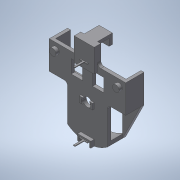
# Autodesk Inventor part: cr2032
Saved by Autodesk Inventor 2021 (Build 250183000, 183)
## iProperties
Created: 2016-08-23
Part Number: cr2032
Material: Generic
Document SubType Name: Modeling
Designer: Federico
Density: 1 g/cm^3
Appearance: Default
Author: Federico
Autodesk Inventor part; units mm, degrees
ref_plane "YZ Plane" through (0, 0, 0) normal (1, 0, 0) x (0, 1, 0)
ref_plane "XZ Plane" through (0, 0, 0) normal (0, 1, 0) x (-1, 0, 0)
ref_plane "XY Plane" through (0, 0, 0) normal (0, 0, 1) x (1, 0, 0)
sketch "Sketch1" plane through (0, 0, 0) normal (0, 1, 0) x (-1, 0, 0)
  line L0 (-2.2802, 25.7355) -> (0.7198, 25.7355)
  line L1 (0.7198, 25.7355) -> (0.7198, 20.2355)
  line L2 (0.7198, 20.2355) -> (9.2198, 20.2355)
  line L3 (9.2198, 20.2355) -> (9.2198, 11.7355)
  line L4 (9.2198, 11.7355) -> (3.7198, 11.7355)
  line L5 (3.7198, 11.7355) -> (3.7198, 0.7355)
  arc A0 (-2.2802, -1.2645) -> (3.7198, 0.7355) centre (-2.2802, 8.7355) ccw
  line L6 (-2.2802, 25.7355) -> (-2.2802, -1.2645)
  point P0 (0, 0)
  dimension "d0" = 3
  dimension "d3" = 8.5
  dimension "d4" = 5.5
  dimension "d5" = 11.5
  dimension "d6" = 6
  dimension "d9" = 27
  dimension "d10" = 11
  constraints: 14 end point, 3 parallel, 3 perpendicular, 2 point on circle, 1 centre point, 1 horizontal, 1 point on line
  measures "d0" distance of L0.start L0.end
  measures "d3" distance of L2.end L3.end
  measures "d4" distance between parallel lines of L2 L0
  measures "d5" distance from line of L3 L0.start
  measures "d6" distance from line of L6.end L5
  measures "d9" distance of L0.start L6.end
  measures "d10" distance of L4.end L5.end
extrude "base" add sketch "Sketch1" along normal blind 1
sketch "Sketch2" plane through (0, 1, 0) normal (0, 1, 0) x (1, 0, 0)
  line L0 (-0.7198, -25.7355) -> (2.2802, -25.7355) projected
  line L1 (2.2802, -25.7355) -> (2.2802, 1.2645) projected
  arc A0 (2.2802, 1.2645) -> (-3.7198, -0.7355) centre (2.2802, -8.7355) ccw projected
  line L2 (-3.7198, -0.7355) -> (-3.7198, -11.7355) projected
  line L3 (-3.7198, -11.7355) -> (-9.2198, -11.7355) projected
  line L4 (-9.2198, -11.7355) -> (-9.2198, -20.2355) projected
  line L5 (-9.2198, -20.2355) -> (-0.7198, -20.2355) projected
  line L6 (-8.3198, -20.2355) -> (-8.3198, -11.7355)
  arc A1 (2.2802, 1.2645) -> (-3.7198, -0.7355) centre (2.2802, -8.7355) ccw
  arc A2 (2.2802, 0.3645) -> (-3.7198, -1.8937) centre (2.2802, -8.7355) ccw
  line L7 (2.2802, -25.7355) -> (0.2802, -25.7355)
  line L8 (0.2802, -25.7355) -> (0.2802, -24.8355)
  line L9 (0.2802, -24.8355) -> (2.2802, -24.8355)
  line L10 (2.2802, -24.8355) -> (2.2802, -25.7355)
  point P0 (0, 0)
  dimension "d13" = 0.9
  dimension "d14" = 0.9
  dimension "d15" = 0.9
  dimension "d16" = 2
  constraints: 10 end point, 4 point on circle, 4 point on line, 2 centre point, 2 concentric, 2 parallel, 2 perpendicular, 1 coincident, 1 horizontal
  measures "d13" radial gap between concentric circles of A0 A2
  measures "d14" distance between parallel lines of L4 L6
  measures "d15" distance between parallel lines of L0 L9
  measures "d16" distance between parallel lines of L1 L8
extrude "sides" add sketch "Sketch2" along normal blind 3.5
sketch "Sketch3" plane through (0, 4.5, 0) normal (0, 1, 0) x (1, 0, 0)
  line L0 (-9.2198, -11.7355) -> (-9.2198, -20.2355) projected
  line L1 (-8.3198, -20.2355) -> (-8.3198, -11.7355) projected
  line L2 (-8.3198, -11.7355) -> (-9.2198, -11.7355) projected
  line L3 (-8.3198, -11.7355) -> (-8.3198, -20.2355) projected
  line L4 (-8.3198, -20.2355) -> (-9.2198, -20.2355) projected
  line L5 (-9.2198, -20.2355) -> (-9.2198, -11.7355) projected
  line L6 (-9.2198, -11.7355) -> (-8.3198, -11.7355) projected
  arc A0 (2.2802, 0.3645) -> (-3.7198, -1.8937) centre (2.2802, -8.7355) ccw projected
  line L7 (-3.7198, -1.8937) -> (-3.7198, -0.7355) projected
  arc A1 (2.2802, 1.2645) -> (-3.7198, -0.7355) centre (2.2802, -8.7355) ccw projected
  line L8 (2.2802, 1.2645) -> (2.2802, 0.3645) projected
  line L9 (0.2802, -25.7355) -> (0.2802, -24.8355) projected
  line L10 (0.2802, -24.8355) -> (2.2802, -24.8355) projected
  line L11 (2.2802, -24.8355) -> (2.2802, -25.7355) projected
  line L12 (2.2802, -25.7355) -> (0.2802, -25.7355) projected
  line L13 (-3.7198, -0.7355) -> (-9.2198, -11.7355)
  line L14 (-3.7198, -1.8937) -> (-3.7198, -9.2355)
  line L15 (-4.7198, -10.2355) -> (-6.8198, -10.2355)
  line L16 (-8.3198, -11.7355) -> (-8.3198, -11.7355)
  line L17 (-3.7198, -11.7355) -> (-8.3198, -11.7355) projected
  arc A2 (-6.8198, -10.2355) -> (-8.3198, -11.7355) centre (-6.8198, -11.7355) ccw
  arc A3 (-4.7198, -10.2355) -> (-3.7198, -9.2355) centre (-4.7198, -9.2355) ccw
  line L18 (2.2802, -25.7355) -> (0.2802, -25.7355)
  line L19 (0.2802, -25.7355) -> (0.2802, -22.7355)
  line L20 (0.2802, -22.7355) -> (2.2802, -22.7355)
  line L21 (2.2802, -22.7355) -> (2.2802, -25.7355)
  point P0 (0, 0)
  point P1 (-8.3198, -10.2355)
  dimension "d19" = 1.5
  dimension "d20" = 1.5
  dimension "d21" = 1
  dimension "d23" = 3
  constraints: 16 end point, 4 point on circle, 4 tangent, 3 perpendicular, 3 point on line, 2 centre point, 2 parallel, 1 collinear, 1 horizontal
  measures "d19" distance between parallel lines of L17 L15
  measures "d20" radius of A2
  measures "d21" radius of A3
  measures "d23" distance between parallel lines of L20 L12
extrude "ceil" add sketch "Sketch3" along normal blind 1
sketch "Sketch6" plane through (0, 0, 0) normal (0, -1, 0) x (1, 0, 0)
  line L0 (-0.7198, 20.2355) -> (-9.2198, 20.2355) projected
  line L1 (-9.2198, 20.2355) -> (-9.2198, 11.7355) projected
  arc A0 (-3.7198, 0.7355) -> (2.2802, -1.2645) centre (2.2802, 8.7355) ccw projected
  line L2 (2.2802, -1.2645) -> (2.2802, 25.7355) projected
  circle A1 centre (-7.2198, 18.2355) radius 1
  line L3 (2.2802, 25.7355) -> (-0.7198, 25.7355)
  line L4 (-0.7198, 25.7355) -> (-0.7198, 18.7355)
  line L5 (-0.7198, 18.7355) -> (2.2802, 18.7355)
  line L6 (2.2802, 18.7355) -> (2.2802, 25.7355)
  line L7 (2.2802, 0.7355) -> (0.2802, 0.7355)
  line L8 (0.2802, 0.7355) -> (0.2802, -1.0625)
  point P0 (0, 0)
  dimension "d26" = 2
  dimension "d27" = 2
  dimension "d28" = 2
  dimension "d29" = 7
  dimension "d30" = 2
  dimension "d31" = 2
  constraints: 12 end point, 3 perpendicular, 2 parallel, 1 centre point, 1 horizontal, 1 point on circle, 1 point on line
  measures "d26" distance from line of L0 A1.centre
  measures "d27" distance from line of L1 A1.centre
  measures "d28" diameter of A1
  measures "d29" distance between parallel lines of L3 L5
  measures "d30" distance from line of L7 L2.start
  measures "d31" distance of L7.start L7.end
extrude "base_separation" add sketch "Sketch6" along normal blind 1
fillet "base_fillet" radius 1 2 edges at (-3.7198, 0.5, 11.7355) (-0.7198, 0.5, 20.2355)
sketch "Sketch7" plane through (0, -1, 0) normal (0, -1, 0) x (1, 0, 0)
  line L0 (2.2802, -1.2645) -> (2.2802, 0.7355) projected
  line L1 (2.2802, 0.1855) -> (1.0302, 0.1855)
  line L2 (1.0302, 0.1855) -> (1.0302, -0.0145)
  line L3 (1.0302, -0.0145) -> (2.2802, -0.0145)
  line L4 (2.2802, -0.0145) -> (2.2802, 0.1855)
  line L5 (2.2802, 20.6855) -> (1.0302, 20.6855)
  line L6 (1.0302, 20.6855) -> (1.0302, 20.4855)
  line L7 (1.0302, 20.4855) -> (2.2802, 20.4855)
  line L8 (2.2802, 20.4855) -> (2.2802, 20.6855)
  line L9 (2.2802, 25.7355) -> (-0.7198, 25.7355) projected
  point P0 (0, 0)
  dimension "d35" = 0.2
  dimension "d37" = 0.2
  dimension "d38" = 20.5
  dimension "d40" = 1.25
  dimension "d41" = 1.25
  dimension "d42" = 1.25
  constraints: 16 end point, 4 parallel, 2 horizontal, 2 perpendicular, 2 point on line
  measures "d35" distance of L7.end L5.start
  measures "d37" distance of L1.end L2.end
  measures "d38" distance between parallel lines of L7 L3
  measures "d40" distance from line of L3 L0.start
  measures "d41" distance of L5.start L5.end
  measures "d42" distance of L2.end L3.end
extrude "pin_base" add sketch "Sketch7" along normal blind 0.25
sketch "Sketch9" plane through (0, -1.25, 0) normal (0, -1, 0) x (1, 0, 0)
  line L0 (1.0302, 20.6855) -> (2.2802, 20.6855) projected
  line L1 (1.0302, 20.4855) -> (2.2802, 20.4855) projected
  line L2 (2.2802, 20.6855) -> (2.0302, 20.6855)
  line L3 (2.0302, 20.6855) -> (2.0302, 20.4855)
  line L4 (2.0302, 20.4855) -> (2.2802, 20.4855)
  line L5 (2.2802, 20.4855) -> (2.2802, 20.6855)
  line L6 (2.2802, 18.7355) -> (2.2802, 20.4855) projected
  line L7 (2.2802, 0.1855) -> (1.0302, 0.1855) projected
  line L8 (2.2802, 0.1855) -> (2.0302, 0.1855)
  line L9 (2.0302, 0.1855) -> (2.0302, -0.0145)
  line L10 (2.0302, -0.0145) -> (2.2802, -0.0145)
  line L11 (2.2802, -0.0145) -> (2.2802, 0.1855)
  line L12 (1.0302, -0.0145) -> (2.2802, -0.0145) projected
  point P0 (0, 0)
  dimension "d45" = 0.25
  constraints: 16 end point, 4 parallel, 2 collinear, 2 horizontal, 2 perpendicular, 1 point on line
  measures "d45" distance between parallel lines of L6 L3
extrude "pin" add sketch "Sketch9" along normal blind 2.75
sketch "Sketch10" plane through (0, 1, 0) normal (0, 1, 0) x (1, 0, 0)
  line L0 (0.7802, -18.3355) -> (-2.6198, -18.3355)
  line L1 (-2.6198, -18.3355) -> (-2.6198, -14.3355)
  line L2 (-2.6198, -14.3355) -> (0.7802, -14.3355)
  line L3 (0.7802, -14.3355) -> (0.7802, -18.3355)
  line L4 (2.2802, -24.8355) -> (2.2802, 0.3645) projected
  line L5 (0.2802, -25.7355) -> (2.2802, -25.7355) projected
  line L6 (0.9052, -9.2355) -> (2.2802, -9.2355)
  line L7 (2.2802, -9.2355) -> (2.2802, -9.7355)
  line L8 (2.2802, -9.7355) -> (0.9052, -9.7355)
  line L9 (0.9052, -9.7355) -> (0.9052, -9.2355)
  point P0 (0, 0)
  dimension "d48" = 4
  dimension "d49" = 3.4
  dimension "d50" = 1.5
  dimension "d51" = 7.4
  dimension "d52" = 16
  dimension "d53" = 16.5
  dimension "d54" = 1.375
  constraints: 16 end point, 4 parallel, 2 horizontal, 2 perpendicular, 1 collinear
  measures "d48" distance of L0.end L1.end
  measures "d49" distance of L0.start L0.end
  measures "d50" distance between parallel lines of L4 L3
  measures "d51" distance between parallel lines of L0 L5
  measures "d52" distance between parallel lines of L8 L5
  measures "d53" distance between parallel lines of L6 L5
  measures "d54" distance of L6.start L6.end
extrude "slot_big" cut sketch "Sketch10" against normal blind 1
sketch "Sketch11" plane through (0, 0, 0) normal (0, -1, 0) x (1, 0, 0)
  line L0 (2.2802, 9.2355) -> (2.2802, -0.3645) projected
  line L1 (2.2802, 9.2355) -> (2.2802, 8.6105)
  line L2 (0.2802, 8.6105) -> (0.2802, 10.3605)
  line L3 (0.2802, 10.3605) -> (2.2802, 10.3605)
  line L4 (2.2802, 24.8355) -> (2.2802, 9.7355) projected
  line L5 (0.9052, 9.7355) -> (2.2802, 9.7355) projected
  line L6 (2.2802, 9.7355) -> (0.9052, 9.7355)
  line L7 (0.9052, 9.2355) -> (0.9052, 9.7355) projected
  line L8 (0.9052, 9.7355) -> (0.9052, 9.2355)
  line L9 (2.2802, 9.2355) -> (0.9052, 9.2355) projected
  line L10 (0.9052, 9.2355) -> (2.2802, 9.2355)
  line L11 (2.2802, 8.6105) -> (0.2802, 8.6105)
  point P0 (0, 0)
  dimension "d59" = 0.625
  dimension "d60" = 2
  dimension "d61" = 0.625
  constraints: 14 end point, 2 collinear, 2 perpendicular, 2 point on line, 1 horizontal, 1 vertical
  measures "d59" distance between parallel lines of L11 L9
  measures "d60" distance between parallel lines of L2 L0
  measures "d61" distance between parallel lines of L5 L3
extrude "slot_small" add sketch "Sketch11" along normal blind 0.5
sketch "Sketch12" plane through (0, 1, 0) normal (0, 1, 0) x (1, 0, 0)
  line L0 (2.2802, -0.7355) -> (2.2802, -8.6105) projected
  arc A0 (2.2802, -1.2355) -> (2.2802, -2.2355) centre (2.2802, -1.7355) ccw
  line L1 (2.2802, -1.2355) -> (2.2802, -2.2355)
  point P0 (0, 0)
  point P1 (2.2802, 1.2645)
  dimension "d64" = 1
  dimension "d65" = 3
  constraints: 3 point on line, 2 end point, 2 point on circle, 1 centre point
  measures "d64" diameter of A0
  measures "d65" distance of point (2.28, 1.265) A0.centre
extrude "tower" add sketch "Sketch12" along normal blind 2.25
sketch "Sketch14" plane through (0, 1, 0) normal (0, 1, 0) x (1, 0, 0)
  circle A0 centre (2.2802, -9.4855) radius 1.375
  line L0 (2.2802, -24.8355) -> (2.2802, -9.7355) projected
  line L1 (2.2802, -9.7355) -> (0.9052, -9.7355) projected
  point P0 (0, 0)
  dimension "d68" = 2.75
  dimension "d69" = 0
  dimension "d70" = 0.25
  constraints: 1 centre point
  measures "d68" diameter of A0
  measures "d69" distance from line of L0 A0.centre
  measures "d70" distance from line of A0.centre L1
extrude "perforacion_2.75" cut sketch "Sketch14" against normal blind 1.5
ref_plane "hole_work_plane" through (2.2802, 0, -1.2645) normal (0, 0, 1) x (0, -1, 0)
sketch "Sketch15" plane through (2.2802, 0, -1.2645) normal (0, 0, 1) x (0, -1, 0)
  line L0 (1, 0) -> (4, 0) projected
  circle A0 centre (1, 0) radius 1.625
  point P0 (0, -2.2802)
  dimension "d74" = 3.25
  constraints: 1 centre point
  measures "d74" diameter of A0
extrude "hole_side_0000" cut sketch "Sketch15" along normal blind 1.25
sketch "Sketch16" plane through (1.0302, -1.25, -0.0145) normal (0, 0, -1) x (-1, 0, 0)
  line L0 (0.375, 0.25) -> (0, 0.25) projected
  arc A0 (0.375, 0.25) -> (-1.25, 1.875) centre (-1.25, 0.25) ccw projected
  arc A1 (0.375, 0.25) -> (0, 1.2883) centre (-1.25, 0.25) ccw
  line L1 (0, 0.25) -> (0, 1.2883)
  point P0 (1.0302, 1.25)
  point P1 (0, 1.2883)
  constraints: 2 end point, 2 point on circle, 1 centre point, 1 concentric, 1 vertical
extrude "hole_side_0001" cut sketch "Sketch16" against normal blind 0.2
mirror "mirror" about plane through (2.2802, 0, 25.7355) normal (1, 0, 0) of "base", "sides", "ceil", "base_separation", "base_fillet", "pin_base", "pin", "slot_big", "slot_small", "tower", "hole_side_0000", "hole_side_0001", "perforacion_2.75"
body "Solid1"
